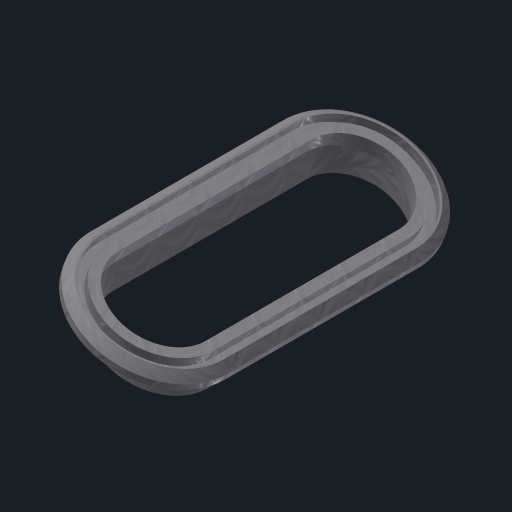
# Autodesk Inventor part: COMPUERTA_PLASTICO
Saved by Autodesk Inventor 2024.3 (Build 283343000, 343)
## iProperties
Created: 2024-07-04
Part Number: COMPUERTA_PLASTICO
Material: Steel, Mild, Welded
Document SubType Name: Modeling
Designer: Niler
Density: 7.85 g/cm^3
Appearance: Weld - Steel Mild
Author: Niler
Autodesk Inventor part; units mm, degrees
ref_plane "YZ Plane" through (0, 0, 0) normal (1, 0, 0) x (0, 1, 0)
ref_plane "XZ Plane" through (0, 0, 0) normal (0, 1, 0) x (-1, 0, 0)
ref_plane "XY Plane" through (0, 0, 0) normal (0, 0, 1) x (1, 0, 0)
sketch "Sketch1" plane through (0, 0, 0) normal (0, 1, 0) x (-1, 0, 0)
  line L0 (-101.5312, 175) -> (101.5312, 175)
  line L1 (101.5312, 175) -> (101.5312, -175)
  line L2 (101.5312, -175) -> (-101.5312, -175)
  line L3 (-101.5312, -175) -> (-101.5312, 175)
  line L4 (-101.5312, 175) -> (101.5312, -175) construction
  line L5 (101.5312, 175) -> (-101.5312, -175) construction
  point P0 (0, 0)
  dimension "d2" = 350
  constraints: 12 end point, 2 midpoint, 2 parallel, 1 horizontal, 1 perpendicular
  measures "d2" distance of L0.end L1.end
extrude "Extrusion1" add sketch "Sketch1" against normal blind 150
sketch "Sketch3" plane through (-101.5312, 0, 175) normal (0, 0, 1) x (-1, 0, 0)
  line L0 (0, 0) -> (-203.0624, 0) projected
  line L1 (-203.0624, 0) -> (-203.0624, 150) projected
  line L2 (-203.0624, 150) -> (0, 150) projected
  line L3 (0, 0) -> (0, 150) projected
  line L4 (0, 150) -> (-48.8156, 150)
  line L5 (0, 0) -> (47.3608, 0)
  line L6 (0, 0) -> (-203.0624, 81.2192)
  point P0 (-101.5312, 0)
  dimension "d7" = 158.2
  constraints: 6 end point, 2 horizontal, 1 point on line
  measures "d7" angle of L5 L6
extrude "Extrusion2" cut sketch "Sketch3" against normal through all contours L0 L1 L6
sketch "Sketch5" plane through (-101.5312, -150, 175) normal (0, 0, 1) x (1, 0, 0)
  line L0 (203.0624, 68.7808) -> (0, 150) projected
  line L1 (203.0624, 44.0093) -> (0, 125.2285)
  line L2 (0, 150) -> (0, 125.2285)
  line L3 (0, 150) -> (0, 0) projected
  line L4 (203.0624, 68.7808) -> (203.0624, 44.0093)
  line L5 (203.0624, 68.7808) -> (203.0624, 0) projected
  line L6 (203.0624, 0) -> (0, 0) projected
  point P0 (101.5312, 150)
  dimension "d13" = 23
  constraints: 8 end point, 1 parallel, 1 point on line, 1 vertical
  measures "d13" distance between parallel lines of L0 L1
extrude "Extrusion4" cut sketch "Sketch5" against normal through all contours L5 L6 L3 L1
sketch "Sketch4" plane through (0, 0, 0) normal (0, 1, 0) x (-1, 0, 0)
  line L0 (0, 100) -> (0, -100) construction
  line L1 (-52.5, 100) -> (-52.5, -100)
  line L2 (52.5, -100) -> (52.5, 100)
  arc A0 (52.5, 100) -> (-52.5, 100) centre (0, 100) ccw
  arc A1 (-52.5, -100) -> (52.5, -100) centre (0, -100) ccw
  line L3 (101.5312, -175) -> (-101.5312, -175) projected
  line L4 (101.5312, -175) -> (101.5312, 175) projected
  line L5 (-101.5312, 175) -> (101.5312, 175) projected
  line L6 (-101.5312, -175) -> (-101.5312, 175) projected
  line L7 (45, -100) -> (45, 100)
  arc A2 (45, 100) -> (-45, 100) centre (0, 100) ccw
  line L8 (-45, 100) -> (-45, -100)
  arc A3 (-45, -100) -> (45, -100) centre (0, -100) ccw
  point P0 (0, 0)
  dimension "d9" = 200
  dimension "d10" = 105
  dimension "d16" = 90
  constraints: 12 end point, 8 point on circle, 4 centre point, 4 tangent, 2 parallel, 1 midpoint, 1 vertical, 3 other
  measures "d9" distance of L0.start L0.end
  measures "d10" distance between parallel lines of L1 L2
  measures "d16" distance between parallel lines of L8 L7
extrude "Extrusion3" cut sketch "Sketch4" against normal through all
sketch "Sketch6" plane through (-52.5, -19.6111, 100) normal (0.3713678, 0.9284858, 0) x (0.9284858, -0.3713678, 0)
  line L0 (0, 200) -> (0, 0) projected
  ellipse E0 centre (56.5437, 0) end of major axis (113.0873, 0) minor radius 52.5 (0, 0) -> (113.0873, 0) ccw projected
  line L1 (113.0873, 0) -> (113.0873, 200) projected
  ellipse E1 centre (56.5437, 200) end of major axis (0, 200) minor radius 52.5 (113.0873, 200) -> (0, 200) ccw projected
  line L2 (105.0097, 200) -> (105.0097, 0) projected
  ellipse E2 centre (56.5437, 0) end of major axis (8.0777, 0) minor radius 45 (8.0777, 0) -> (105.0097, 0) ccw projected
  line L3 (8.0777, 0) -> (8.0777, 200) projected
  ellipse E3 centre (56.5437, 200) end of major axis (105.0097, 200) minor radius 45 (105.0097, 200) -> (8.0777, 200) ccw projected
  line L4 (-20, 0) -> (-20, 200)
  line L5 (133.0873, 200) -> (133.0873, 0)
  spline S0 degree 5 poles (-20, 200) (-20, 203.1018) (-19.8251, 206.2037) (-19.4753, 209.2923) (-17.2468, 222.3406) (-11.946, 234.687) (-6.2162, 243.2846) (7.9884, 258.1937) (26.2772, 267.6785) (36.1418, 270.8912) (56.5437, 274.109) (76.9455, 270.8912) (86.8102, 267.6785) (105.0989, 258.1937) (119.3036, 243.2846) (125.0334, 234.687) (130.3341, 222.3406) (132.5626, 209.2923) (132.9125, 206.2037) (133.0874, 203.1018) (133.0873, 200) knots 0 0 0 0 0 0 0.066229 0.066229 0.066229 0.282193 0.282193 0.282193 0.5 0.5 0.5 0.717807 0.717807 0.717807 0.933771 0.933771 0.933771 1 1 1 1 1 1
  spline S1 degree 5 poles (133.0873, 0) (133.0874, -3.1018) (132.9125, -6.2037) (132.5626, -9.2923) (130.3341, -22.3406) (125.0334, -34.687) (119.3036, -43.2846) (105.0989, -58.1937) (86.8102, -67.6785) (76.9455, -70.8912) (56.5437, -74.109) (36.1418, -70.8912) (26.2772, -67.6785) (7.9884, -58.1937) (-6.2162, -43.2846) (-11.946, -34.687) (-17.2468, -22.3406) (-19.4753, -9.2923) (-19.8251, -6.2037) (-20, -3.1018) (-20, 0) knots 0 0 0 0 0 0 0.066229 0.066229 0.066229 0.282193 0.282193 0.282193 0.5 0.5 0.5 0.717807 0.717807 0.717807 0.933771 0.933771 0.933771 1 1 1 1 1 1
  point P0 (41.4626, 100)
  dimension "d17" = 20
  constraints: 4 end point, 3 parallel, 2 horizontal alignment, 8 other
  measures "d17" distance between parallel lines of L0 L4
extrude "Extrusion5" add sketch "Sketch6" along normal blind 15 contours E1 L1 E0 L0 | L4 S0 L5 S1
sketch "Sketch7" plane through (-46.9295, -5.6838, 100) normal (0.3713678, 0.9284858, 0) x (0.9284858, -0.3713678, 0)
  line L0 (133.0873, 0) -> (133.0873, 200) projected
  spline S0 degree 5 poles (133.0873, 200) (133.0874, 203.1018) (132.9125, 206.2037) (132.5626, 209.2923) (130.3341, 222.3406) (125.0334, 234.687) (119.3036, 243.2846) (105.0989, 258.1937) (86.8102, 267.6785) (76.9455, 270.8912) (56.5437, 274.109) (36.1418, 270.8912) (26.2772, 267.6785) (7.9884, 258.1937) (-6.2162, 243.2846) (-11.946, 234.687) (-17.2468, 222.3406) (-19.4753, 209.2923) (-19.8251, 206.2037) (-20, 203.1018) (-20, 200) knots 0 0 0 0 0 0 0.066229 0.066229 0.066229 0.282193 0.282193 0.282193 0.5 0.5 0.5 0.717807 0.717807 0.717807 0.933771 0.933771 0.933771 1 1 1 1 1 1
  line L1 (-20, 200) -> (-20, 0) projected
  spline S1 degree 5 poles (-20, 0) (-20, -3.1018) (-19.8251, -6.2037) (-19.4753, -9.2923) (-17.2468, -22.3406) (-11.946, -34.687) (-6.2162, -43.2846) (7.9884, -58.1937) (26.2772, -67.6785) (36.1418, -70.8912) (56.5437, -74.109) (76.9455, -70.8912) (86.8102, -67.6785) (105.0989, -58.1937) (119.3036, -43.2846) (125.0334, -34.687) (130.3341, -22.3406) (132.5626, -9.2923) (132.9125, -6.2037) (133.0874, -3.1018) (133.0873, 0) knots 0 0 0 0 0 0 0.066229 0.066229 0.066229 0.282193 0.282193 0.282193 0.5 0.5 0.5 0.717807 0.717807 0.717807 0.933771 0.933771 0.933771 1 1 1 1 1 1
  line L2 (8.0777, 0) -> (8.0777, 200) projected
  ellipse E0 centre (56.5437, 200) end of major axis (8.0777, 200) minor radius 45 (105.0097, 200) -> (8.0777, 200) ccw projected
  line L3 (105.0097, 200) -> (105.0097, 0) projected
  ellipse E1 centre (56.5437, 0) end of major axis (105.0097, 0) minor radius 45 (8.0777, 0) -> (105.0097, 0) ccw projected
  line L4 (123.0873, 0) -> (123.0873, 200)
  line L5 (-10, 200) -> (-10, 0)
  line L6 (115.0097, 0) -> (115.0097, 200)
  line L7 (-1.9223, 200) -> (-1.9223, 0)
  spline S2 degree 5 poles (123.0873, 200.0001) (123.0872, 208.0319) (121.7154, 216.066) (118.9663, 223.781) (110.9834, 238.082) (98.9156, 249.1661) (92.0237, 253.7365) (77.051, 260.7114) (60.7013, 263.0958) (52.386, 263.0958) (36.0363, 260.7114) (21.0636, 253.7365) (14.1717, 249.1661) (2.104, 238.082) (-5.879, 223.781) (-8.628, 216.066) (-9.9999, 208.032) (-10, 200.0002) knots 0 0 0 0 0 0 0.198071 0.198071 0.198071 0.398853 0.398853 0.398853 0.601147 0.601147 0.601147 0.801929 0.801929 0.801929 1 1 1 1 1 1
  spline S3 degree 5 poles (-10, -0.0001) (-9.9999, -8.0319) (-8.628, -16.066) (-5.879, -23.781) (2.104, -38.082) (14.1717, -49.1661) (21.0636, -53.7365) (36.0363, -60.7114) (52.386, -63.0958) (60.7013, -63.0958) (77.051, -60.7114) (92.0237, -53.7365) (98.9156, -49.1661) (110.9834, -38.082) (118.9663, -23.781) (121.7154, -16.066) (123.0872, -8.0319) (123.0873, -0.0001) knots 0 0 0 0 0 0 0.198071 0.198071 0.198071 0.398853 0.398853 0.398853 0.601147 0.601147 0.601147 0.801929 0.801929 0.801929 1 1 1 1 1 1
  spline S4 degree 5 poles (115.0097, 200) (115.0097, 202.3372) (114.8779, 204.6744) (114.6142, 207.0017) (112.9267, 216.8797) (108.904, 226.2243) (104.5495, 232.7355) (93.7083, 244.0903) (79.7551, 251.3124) (72.189, 253.7694) (56.5437, 256.2308) (40.8983, 253.7694) (33.3322, 251.3124) (19.379, 244.0903) (8.5379, 232.7355) (4.1833, 226.2243) (0.1606, 216.8797) (-1.5268, 207.0017) (-1.7905, 204.6744) (-1.9224, 202.3372) (-1.9223, 200) knots 0 0 0 0 0 0 0.065549 0.065549 0.065549 0.280608 0.280608 0.280608 0.5 0.5 0.5 0.719392 0.719392 0.719392 0.934451 0.934451 0.934451 1 1 1 1 1 1
  spline S5 degree 5 poles (-1.9223, 0) (-1.9224, -2.3372) (-1.7905, -4.6744) (-1.5268, -7.0017) (0.1606, -16.8797) (4.1833, -26.2243) (8.5379, -32.7355) (19.379, -44.0903) (33.3322, -51.3124) (40.8983, -53.7694) (56.5437, -56.2308) (72.189, -53.7694) (79.7551, -51.3124) (93.7083, -44.0903) (104.5495, -32.7355) (108.904, -26.2243) (112.9267, -16.8797) (114.6142, -7.0017) (114.8779, -4.6744) (115.0097, -2.3372) (115.0097, 0) knots 0 0 0 0 0 0 0.065549 0.065549 0.065549 0.280608 0.280608 0.280608 0.5 0.5 0.5 0.719392 0.719392 0.719392 0.934451 0.934451 0.934451 1 1 1 1 1 1
  point P0 (41.4626, 100)
  dimension "d20" = 10
  dimension "d21" = 10
  constraints: 8 end point, 6 horizontal alignment, 6 parallel, 10 other
extrude "Extrusion6" cut sketch "Sketch7" against normal blind 10 contours S3 L5 S2 L4
chamfer "Chamfer1" distance 8 angle 45 4 edges at (5.5705, -26.6823, 172.5001) (76.6402, -55.1081, 0) (5.5705, -26.6823, -172.5001) (-65.4992, 1.7436, 0)
body "Solid1"
